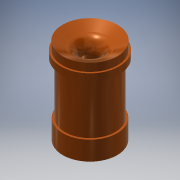
# Autodesk Inventor part: Phenolic 8-inch v1
Saved by Autodesk Inventor 2017 (Build 210142000, 142)
## iProperties
Created: 2016-01-09
Part Number: Phenolic 8-inch v1
Material: Phenolic Resin
Document SubType Name: Modeling
Designer: Jared
Density: 1.38 g/cm^3
Appearance: Smooth - Light Orange
Author: Jared
Autodesk Inventor part; units mm, degrees
ref_plane "YZ Plane" through (0, 0, 0) normal (1, 0, 0) x (0, 1, 0)
ref_plane "XZ Plane" through (0, 0, 0) normal (0, 1, 0) x (-1, 0, 0)
ref_plane "XY Plane" through (0, 0, 0) normal (0, 0, 1) x (1, 0, 0)
sketch "Sketch1" plane through (0, 0, 0) normal (0, 0, 1) x (1, 0, 0)
  arc A0 (-25.8327, -3.287) -> (-25.4, 0) centre (-38.1, 0) ccw
  line L0 (-25.8327, -3.287) -> (-64.6621, -148.2003)
  line L1 (-87.8501, 55.3459) -> (-87.8501, 29.9459)
  line L2 (-87.8501, 29.9459) -> (-93.4, 29.9459)
  line L3 (-59.2667, 42.6459) -> (-60.6149, 42.6459)
  line L4 (-59.2667, 42.6459) -> (0, 42.6459) construction
  line L5 (-41.4694, -37.9453) -> (-35.1194, -37.9453)
  line L6 (-93.4, 29.9459) -> (-93.4, 17.2459)
  line L7 (-93.4, 17.2459) -> (-80.7, 17.2459)
  line L8 (-80.7, 17.2459) -> (-74.35, 17.2459)
  line L9 (-74.35, 17.2459) -> (-74.35, -160.6575)
  line L10 (-93.4, 17.2459) -> (-93.4, 7.7209)
  line L11 (-93.4, 17.2459) -> (-83.875, 17.2459) construction
  line L12 (-93.4, 7.7209) -> (-80.7, 7.7209)
  line L13 (-80.7, 7.7209) -> (-80.7, -43.0791)
  line L14 (-80.7, -43.0791) -> (-93.4, -43.0791)
  line L15 (-93.4, 7.7209) -> (-87.05, 7.7209)
  line L16 (-87.05, 7.7209) -> (-87.05, 1.7773)
  line L17 (-87.05, 1.7773) -> (-93.4, 1.7773)
  line L18 (-93.4, 29.9459) -> (-93.4, 7.7209)
  line L19 (-93.4, 1.7773) -> (-93.4, -43.0791)
  line L20 (-80.7, -43.0791) -> (-80.7, -184.356)
  line L21 (-80.7, -43.0791) -> (-21.9625, -43.0791) construction
  line L22 (-68, -160.6575) -> (-74.35, -160.6575)
  line L23 (-87.05, -109.8575) -> (-80.7, -109.8575)
  line L24 (-64.6621, -148.2003) -> (-83.875, -219.9038)
  line L25 (-64.6621, -148.2003) -> (-40.1276, -148.2003) construction
  line L26 (-87.05, -219.9038) -> (-83.875, -219.9038)
  line L27 (-80.7, -184.356) -> (-74.35, -184.356)
  line L28 (0, 42.6459) -> (0, 0)
  line L29 (-87.05, -158.956) -> (-87.05, -219.9038)
  line L30 (-80.7, -109.8575) -> (-83.875, -109.8575)
  line L31 (-87.05, -158.956) -> (-80.7, -158.956)
  line L32 (-87.8501, 55.3459) -> (-18.3062, 55.3459) construction
  line L33 (-87.8501, 55.3459) -> (-14.7047, 55.3459) construction
  line L34 (-87.8501, 55.3459) -> (-55.5582, 40.2879)
  line L35 (-87.8501, 55.3459) -> (-52.22, 55.3459) construction
  arc A1 (-25.4, 0) -> (-55.5582, 40.2879) centre (-67.3891, 0) ccw
  line L36 (-59.2667, 42.6459) -> (-59.2667, -37.9453)
  line L37 (-59.2667, 42.6459) -> (21.3245, 42.6459) construction
  line L38 (-59.2667, -37.9453) -> (-41.4694, -37.9453)
  dimension "d86" = 25.4
  dimension "d87" = 25.4
  dimension "d88" = 5.5499
  dimension "d89" = 87.8501
  dimension "d90" = 12.7
  dimension "d91" = 12.7
  dimension "d92" = 59.2667
  dimension "d93" = 6.35
  dimension "d94" = 105
  dimension "d95" = 12.7
  dimension "d96" = 12.7
  dimension "d97" = 6.35
  dimension "d98" = 9.525
  dimension "d99" = 50.8
  dimension "d100" = 12.7
  dimension "d101" = 6.35
  dimension "d102" = 5.9436
  dimension "d103" = 6.35
  dimension "d104" = 50.8
  dimension "d105" = 6.35
  dimension "d106" = 105
  dimension "d107" = 3.175
  dimension "d108" = 6.35
  dimension "d109" = 60.9478
  dimension "d110" = 3.175
  dimension "d111" = 6.35
  dimension "d112" = 25.4
  dimension "d113" = 25
  dimension "d114" = 41.9891
  dimension "d115" = 32.2919
  dimension "d116" = 90
  dimension "d117" = 80.5912
  constraints: 79 end point, 15 perpendicular, 13 horizontal, 8 point on line, 4 point on circle, 4 vertical, 3 equal length, 3 horizontal alignment, 2 centre point, 2 collinear, 2 midpoint, 1 parallel, 1 tangent, 1 vertical alignment, 1 other
  measures "d86" distance of A1.start L28.end
  measures "d87" distance of L1.start L1.end
  measures "d88" distance of L1.end L6.start
  measures "d89" distance from line of L28.end L1
  measures "d90" vertical distance of L3.start L1.start
  measures "d91" radius of A0
  measures "d92" horizontal distance of L28.end L3.start
  measures "d93" distance of L5.start L5.end
  measures "d94" angle of L5 L0
  measures "d95" distance of L6.start L6.end
  measures "d96" distance of L6.end L8.start
  measures "d97" distance of L8.start L9.start
  measures "d98" distance of L6.end L18.end
  measures "d99" distance of L12.end L21.start
  measures "d100" distance of L18.end L12.end
  measures "d101" distance of L18.end L15.end
  measures "d102" distance of L15.end L17.start
  measures "d103" distance of L9.end L22.start
  measures "d104" distance between parallel lines of L22 L23
  measures "d105" distance of L23.start L30.start
  measures "d106" angle of L24 L25
  measures "d107" distance of L24.end L29.end
  measures "d108" distance of L20.end L27.end
  measures "d109" distance of L31.start L29.end
  measures "d110" distance of L30.start L30.end
  measures "d111" distance from line of L20 L31.start
  measures "d112" distance between parallel lines of L31 L27
  measures "d113" angle of L34 L35
  measures "d114" radius of A1
  measures "d115" horizontal distance of L1.start L34.end
  measures "d116" angle of L36 L37
  measures "d117" distance of L3.start L38.start
revolve "Revolution1" add sketch "Sketch1" angle 360 about axis through (0, 42.6459, 0) along (0, -1, 0) contours L0 L5 L38 L36 L34 A1 A0 | L0 L24 L22 L9 L8 L7 L6 L2 L1 L34 L36 L38 L5 | L24 L27 L20 L13 L12 L10 L7 L8 L9 L22 | L24 L26 L29 L31 L20 L27
body "Solid1"
